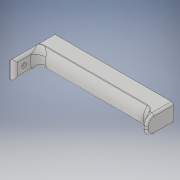
# Autodesk Inventor part: SpoolHolder
Saved by Autodesk Inventor 2018 (Build 220112000, 112)
## iProperties
Created: 2017-10-07
Part Number: SpoolHolder
Material: Generic
Document SubType Name: Modeling
Designer: Jurjen
Density: 1 g/cm^3
Appearance: Default
Author: Jurjen
Autodesk Inventor part; units mm, degrees
ref_plane "YZ Plane" through (0, 0, 0) normal (1, 0, 0) x (0, 1, 0)
ref_plane "XZ Plane" through (0, 0, 0) normal (0, 1, 0) x (-1, 0, 0)
ref_plane "XY Plane" through (0, 0, 0) normal (0, 0, 1) x (1, 0, 0)
sketch "Sketch1" plane through (0, 0, 0) normal (1, 0, 0) x (0, 1, 0)
  line L0 (-8.5, -7) -> (8.5, -7)
  line L1 (8.5, -7) -> (8.5, 7)
  line L2 (-8.5, -7) -> (-8.5, 7)
  arc A0 (8.5, 7) -> (-8.5, 7) centre (0, 0.0179) ccw
  point P0 (0, 0)
  point P1 (0, -7)
  point P2 (8.5, 0)
  dimension "d1" = 17
  dimension "d2" = 14
  dimension "d3" = 11
  constraints: 6 end point, 2 horizontal alignment, 2 midpoint, 2 point on circle, 1 centre point, 1 horizontal, 1 perpendicular, 1 vertical, 1 vertical alignment
  measures "d1" distance between parallel lines of L1 L2
  measures "d2" distance of L0.end L1.end
  measures "d3" radius of A0
extrude "Extrusion1" add sketch "Sketch1" along normal mid plane 105
sketch "Sketch2" plane through (-52.5, 0, 0) normal (-1, 0, 0) x (0, 0, 1)
  line L0 (-7, -8.5) -> (-7, 8.5) projected
  line L1 (-7, 8.5) -> (33, 8.5)
  line L2 (33, 8.5) -> (33, -8.5)
  line L3 (33, -8.5) -> (-7, -8.5)
  line L4 (-7, -8.5) -> (-7, 8.5)
  point P0 (0, 0)
  point P1 (7, -8.5)
  dimension "d6" = 40
  constraints: 8 end point, 2 parallel, 1 horizontal, 1 horizontal alignment, 1 perpendicular
  measures "d6" distance of L2.end L3.end
extrude "Extrusion2" add sketch "Sketch2" along normal blind 4
fillet "Fillet3" radius 3 3 edges at (-52.5, -8.5, 20) (-52.5, 8.5, 20) (-52.5, 0, 33)
fillet "Fillet4" radius 7 3 edges at (-53.3997, 7.6421, 7.9298) (-53.3991, -7.6415, 7.9304) (-52.5, 0, 11.0179)
sketch "Sketch3" plane through (-52.5, 0, 0) normal (1, 0, 0) x (0, 0, -1)
  circle A0 centre (-23.8591, 0) radius 2.1
  point P0 (0, 0)
  dimension "d13" = 4.2
  constraints: 1 centre point
  measures "d13" diameter of A0
extrude "Extrusion3" cut sketch "Sketch3" against normal up to next
sketch "Sketch4" plane through (52.5, 0, 0) normal (1, 0, 0) x (0, 0, -1)
  line L0 (-7, -8.5) -> (7, -8.5) projected
  line L1 (-33, 8.5) -> (7, 8.5) projected
  line L2 (7, -8.5) -> (-18, -8.5)
  line L3 (-18, -8.5) -> (-18, 8.5)
  line L4 (-18, 8.5) -> (7, 8.5)
  line L5 (7, 8.5) -> (7, -8.5)
  point P0 (0, 0)
  dimension "d16" = 25
  constraints: 8 end point, 2 parallel, 1 horizontal, 1 perpendicular, 1 point on line
  measures "d16" distance between parallel lines of L5 L3
extrude "Extrusion4" add sketch "Sketch4" along normal blind 3
fillet "Fillet5" radius 7 3 edges at (52.5, 0, 11.0179) (54, -8.5, 18) (54, 8.5, 18)
fillet "Fillet6" radius 2 5 edges at (55.5, -6.4497, 15.9497) (55.5, 0, 18) (55.5, 6.4497, 15.9497) (55.5, 8.5, 2) (55.5, -8.5, 2)
fillet "Fillet7" radius 1 13 edges at (52.5, 0, 18) (52.5, 1.151, 18) (52.5, 2.663, 17.9027) (52.355, 7.3122, 14.9011) (48.825, 8.5, 8.2604) (-2.2941, 8.5, 7) (-53.307, 8.5, 7.5416) (52.5, -2.663, 17.9027) (52.355, -7.3122, 14.9011) (48.825, -8.5, 8.2604) (-2.2941, -8.5, 7) (-53.307, -8.5, 7.5416) (52.5, -1.151, 18)
sketch "Sketch5" plane through (-56.5, 0, 0) normal (-1, 0, 0) x (0, 0, 1)
  line L0 (-7, 8.5) -> (-7, -8.5) projected
  line L1 (3, 2.5) -> (-7, 2.5)
  line L2 (-7, 2.5) -> (-7, -2.5)
  line L3 (-7, -2.5) -> (3, -2.5)
  line L4 (3, -2.5) -> (3, 2.5)
  point P0 (0, 0)
  point P1 (-7, 0)
  dimension "d22" = 5
  dimension "d23" = 10
  constraints: 8 end point, 2 parallel, 1 horizontal, 1 horizontal alignment, 1 midpoint, 1 perpendicular, 1 point on line
  measures "d22" distance between parallel lines of L3 L1
  measures "d23" distance between parallel lines of L0 L4
extrude "Extrusion5" add sketch "Sketch5" along normal blind 3
chamfer "Chamfer1" distance 2 angle 45 6 edges at (-59.5, -2.5, -2) (-59.5, 2.5, -2) (-56.5, 8.5, 13) (-59.5, 0, 3) (-58, -2.5, 3) (-58, 2.5, 3)
body "Solid1"
